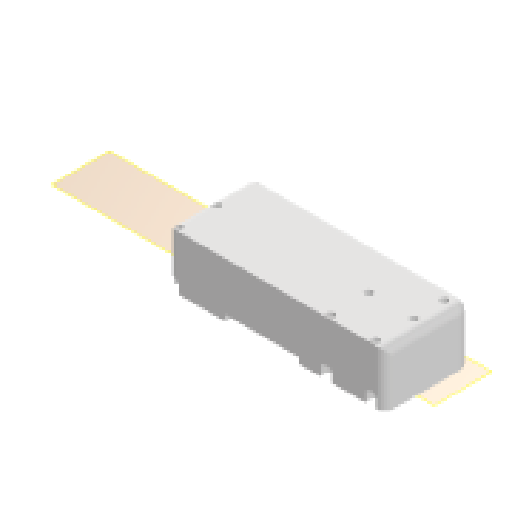
# Autodesk Inventor part: 10_Wellplate_base_Lasercover
Saved by Autodesk Inventor 2024.1 (Build 281209000, 209)
## iProperties
Created: 2024-08-29
Part Number: 10_Wellplate_base_Lasercover
Material: Generisch
Document SubType Name: Modeling
Designer: diederichbenedict
Density: 1 g/cm^3
Appearance: Vorgabe
Author: diederichbenedict
Autodesk Inventor part; units mm, degrees
ref_plane "YZ Plane" through (0, 0, 0) normal (1, 0, 0) x (0, 1, 0)
ref_plane "XZ Plane" through (0, 0, 0) normal (0, 1, 0) x (-1, 0, 0)
ref_plane "XY Plane" through (0, 0, 0) normal (0, 0, 1) x (1, 0, 0)
ref_plane "Arbeitsebene1" through (0, 0, 0) normal (0, 0, 1) x (1, 0, 0)
sketch "Skizze1" plane through (0, 0, 0) normal (0, 0, 1) x (1, 0, 0)
  line L0 (37.9, 26.5) -> (37.9, 13.35) projected
  line L1 (37.9, 13.35) -> (53.9, 13.35) projected
  line L2 (53.9, 13.35) -> (53.9, 13.85) projected
  line L3 (53.9, 13.85) -> (63.9, 13.85) projected
  line L4 (63.9, 13.85) -> (63.9, 27.75) projected
  arc A0 (63.9, 27.75) -> (58.9, 32.75) centre (58.9, 27.75) ccw projected
  line L5 (58.9, 32.75) -> (-58.9, 32.75) projected
  arc A1 (-58.9, 32.75) -> (-63.9, 27.75) centre (-58.9, 27.75) ccw projected
  line L6 (-63.9, 27.75) -> (-63.9, 19.25) projected
  line L7 (-63.9, 19.25) -> (-58.9, 19.25) projected
  line L8 (-58.9, 19.25) -> (-58.9, 19.75) projected
  line L9 (-58.9, 19.75) -> (-38.9, 19.75) projected
  line L10 (-38.9, 19.75) -> (-38.9, 13.85) projected
  line L11 (-38.9, 13.85) -> (-28.9, 13.85) projected
  line L12 (-28.9, 13.85) -> (-28.9, 13.35) projected
  line L13 (-28.9, 13.35) -> (-8.6, 13.35) projected
  line L14 (-8.6, 13.35) -> (-8.6, 26.5) projected
  line L15 (-8.6, 26.5) -> (37.9, 26.5) projected
  circle A2 centre (58.6204, 27.75) radius 1.4 projected
  circle A3 centre (-59.1796, 27.75) radius 1.4 projected
  circle A4 centre (-13.6, 16.25) radius 1.4 projected
  circle A5 centre (-33.6, 16.25) radius 1.4 projected
  circle A6 centre (58.9, 16.25) radius 1.4 projected
  circle A7 centre (42.4, 16.25) radius 1.4 projected
  line L16 (-8.6, -11.9682) -> (-10.6, -13.9682) projected
  line L17 (-8.6, -11.9682) -> (-8.6, 5.15) projected
  line L18 (-8.6, 5.15) -> (-28.9, 5.15) projected
  line L19 (-28.9, 5.15) -> (-28.9, 4.65) projected
  line L20 (-28.9, 4.65) -> (-38.9, 4.65) projected
  line L21 (-38.9, 4.65) -> (-38.9, -1.25) projected
  line L22 (-38.9, -1.25) -> (-58.9, -1.25) projected
  line L23 (-58.9, -1.25) -> (-58.9, -0.75) projected
  line L24 (-58.9, -0.75) -> (-63.9, -0.75) projected
  line L25 (-63.9, -0.75) -> (-63.9, -16.5797) projected
  arc A8 (-49.9, -11.2196) -> (-63.9, -16.5797) centre (-50.2702, -31.2162) ccw projected
  line L26 (-49.9, -11.2196) -> (-49.9, -13.9682) projected
  line L27 (-49.9, -13.9682) -> (-10.6, -13.9682) projected
  circle A9 centre (-13.3796, -11.2637) radius 1.4 projected
  circle A10 centre (-33.6, 2.25) radius 1.4 projected
  circle A11 centre (-13.6, 2.25) radius 1.4 projected
  circle A12 centre (58.6204, -47.75) radius 1.4 projected
  circle A13 centre (58.9, 2.25) radius 1.4 projected
  circle A14 centre (42.4, 2.25) radius 1.4 projected
  circle A15 centre (42.4, -11.2637) radius 1.4 projected
  circle A16 centre (42.4, -31.25) radius 1.4 projected
  line L28 (63.9, 4.65) -> (53.9, 4.65) projected
  line L29 (53.9, 4.65) -> (53.9, 5.15) projected
  line L30 (53.9, 5.15) -> (37.9, 5.15) projected
  line L31 (37.9, 5.15) -> (37.9, -41.35) projected
  line L32 (37.9, -41.35) -> (-33.0276, -41.35) projected
  arc A17 (-59.1255, -49.149) -> (-33.0276, -41.35) centre (-50.2702, -31.2162) ccw projected
  arc A18 (-60.3777, -48.4742) -> (-59.1255, -49.149) centre (-59.1796, -47.75) ccw projected
  arc A19 (-63.9, -45.8527) -> (-60.3777, -48.4742) centre (-50.2702, -31.2162) ccw projected
  line L33 (-63.9, -45.8527) -> (-63.9, -47.75) projected
  arc A20 (-63.9, -47.75) -> (-58.9, -52.75) centre (-58.9, -47.75) ccw projected
  line L34 (-58.9, -52.75) -> (58.9, -52.75) projected
  arc A21 (58.9, -52.75) -> (63.9, -47.75) centre (58.9, -47.75) ccw projected
  line L35 (63.9, -47.75) -> (63.9, 4.65) projected
  line L36 (-16.1, 32.75) -> (63.9, 32.75)
  line L37 (63.9, 32.75) -> (63.9, 0.75)
  line L38 (63.9, 0.75) -> (-16.1, 0.75)
  line L39 (-16.1, 0.75) -> (-16.1, 32.75)
  point P0 (0, 0)
  dimension "d0" = 80
  dimension "d1" = 0
  dimension "d2" = 32
  constraints: 8 end point, 2 parallel, 1 horizontal, 1 perpendicular, 1 point on line
  measures "d0" distance between parallel lines of L4 L39
  measures "d1" distance between parallel lines of L5 L36
  measures "d2" distance between parallel lines of L38 L36
extrude "Extrusion1" add sketch "Skizze1" along normal blind 20 contours L15 L14 L13 L39 L5 A0 L4 L3 L2 L1 L0 | L0 L1 L2 L3 L37 L28 L29 L30 L31 L38 L17 L18 L39 L13 L14 L15 | L18 L17 L38 L39 | L35 L38 L31 L30 L29 L28
fillet "Rundung1" radius 3 9 edges at (62.4355, 31.2855, 20) (63.9, 20.8, 20) (63.9, 9.25, 20) (63.9, 2.7, 20) (21.4, 32.75, 20) (-16.1, 16.75, 20) (-16.1, 0.75, 10) (-16.1, 32.75, 10) (63.9, 0.75, 10)
sketch "Skizze2" plane through (0, 0, 0) normal (0, 0, -1) x (-1, 0, 0)
  arc A0 (13.1, 0.75) -> (16.1, 3.75) centre (13.1, 3.75) ccw projected
  line L0 (16.1, 29.75) -> (16.1, 3.75) projected
  arc A1 (16.1, 29.75) -> (13.1, 32.75) centre (13.1, 29.75) ccw projected
  line L1 (-58.9, 32.75) -> (13.1, 32.75) projected
  arc A2 (-58.9, 32.75) -> (-63.9, 27.75) centre (-58.9, 27.75) ccw projected
  line L2 (-63.9, 3.75) -> (-63.9, 27.75) projected
  arc A3 (-63.9, 3.75) -> (-60.9, 0.75) centre (-60.9, 3.75) ccw projected
  line L3 (13.1, 0.75) -> (-60.9, 0.75) projected
  circle A4 centre (13.6, 2.25) radius 1.4 projected
  circle A5 centre (-42.4, 2.25) radius 1.4 projected
  circle A6 centre (-58.9, 2.25) radius 1.4 projected
  circle A7 centre (-42.4, 16.25) radius 1.4 projected
  circle A8 centre (-58.9, 16.25) radius 1.4 projected
  circle A9 centre (13.6, 16.25) radius 1.4 projected
  circle A10 centre (-58.6204, 27.75) radius 1.4 projected
  point P0 (0, 0)
hole "Bohrung1" at (58.6204, 27.75, 0) at (42.4, 16.25, 0) at (58.9, 2.25, 0) at (58.9, 16.25, 0) at (42.4, 2.25, 0) at (-13.6, 2.25, 0) at (-13.6, 16.25, 0) direction (0, 0, 1) diameter 4.9 depth 4 tip angle 118
sketch "Skizze3" plane through (0, 0, 0) normal (0, 0, -1) x (-1, 0, 0)
  arc A0 (15.9692, 2.8739) -> (11.6629, 0.75) centre (13.6, 2.25) ccw projected
  arc A1 (15.9692, 2.8739) -> (16.1, 3.75) centre (13.1, 3.75) ccw projected
  line L0 (16.1, 29.75) -> (16.1, 3.75) projected
  arc A2 (16.1, 29.75) -> (13.1, 32.75) centre (13.1, 29.75) ccw projected
  line L1 (-58.9, 32.75) -> (13.1, 32.75) projected
  arc A3 (-58.9, 32.75) -> (-63.9, 27.75) centre (-58.9, 27.75) ccw projected
  line L2 (-63.9, 3.75) -> (-63.9, 27.75) projected
  arc A4 (-63.9, 3.75) -> (-60.9, 0.75) centre (-60.9, 3.75) ccw projected
  line L3 (-60.8371, 0.75) -> (-60.9, 0.75) projected
  arc A5 (-56.9629, 0.75) -> (-60.8371, 0.75) centre (-58.9, 2.25) ccw projected
  line L4 (-44.3371, 0.75) -> (-56.9629, 0.75) projected
  arc A6 (-40.4629, 0.75) -> (-44.3371, 0.75) centre (-42.4, 2.25) ccw projected
  line L5 (11.6629, 0.75) -> (-40.4629, 0.75) projected
  circle A7 centre (-58.6204, 27.75) radius 2.45 projected
  circle A8 centre (-42.4, 16.25) radius 2.45 projected
  circle A9 centre (-58.9, 16.25) radius 2.45 projected
  circle A10 centre (13.6, 16.25) radius 2.45 projected
  arc A11 (-58.9, 31.2519) -> (-62.4019, 27.75) centre (-58.9, 27.75) ccw
  line L6 (-58.9, 31.2519) -> (13.1, 31.2519)
  arc A12 (14.6019, 29.75) -> (13.1, 31.2519) centre (13.1, 29.75) ccw
  line L7 (14.6019, 29.75) -> (14.6019, 6.0689)
  arc A13 (14.6019, 6.0689) -> (9.6519, 2.2481) centre (13.6, 2.25) ccw
  line L8 (9.6519, 2.2481) -> (-38.4519, 2.2481)
  arc A14 (-38.4519, 2.2481) -> (-46.3481, 2.2481) centre (-42.4, 2.25) ccw
  line L9 (-46.3481, 2.2481) -> (-54.9519, 2.2481)
  arc A15 (-54.9519, 2.2481) -> (-62.3327, 4.2005) centre (-58.9, 2.25) ccw
  arc A16 (-62.4019, 3.75) -> (-62.3327, 4.2005) centre (-60.9, 3.75) ccw
  line L10 (-62.4019, 3.75) -> (-62.4019, 27.75)
  circle A17 centre (-58.9, 16.25) radius 3.4626
  circle A18 centre (-58.6204, 27.75) radius 3.6913
  circle A19 centre (-42.4, 16.25) radius 3.7166
  circle A20 centre (13.6, 16.25) radius 4.3613
  point P0 (0, 0)
  point P1 (-57.4529, 31.2519)
  point P2 (-61.1978, 30.3926)
  point P3 (-61.3491, 2.3169)
  point P4 (-59.6499, 4.5824)
  point P5 (-61.7336, 4.9993)
  point P6 (14.6019, 12.0053)
  point P7 (14.6019, 20.4947)
  constraints: 12 point on circle, 10 centre point, 10 end point, 10 other
extrude "Extrusion2" cut sketch "Skizze3" against normal blind 18 contours L7 A13 L8 A14 L9 A15 A16 A5 L10 A11 A18 L6 A12 A20
sketch "Skizze4" plane through (-13.1, 0.75, 20) normal (0, -1, 0) x (1, 0, 0)
  circle A0 centre (31.7066, -26.8441) radius 6 projected
  line L0 (45.2066, -35.8441) -> (18.2066, -35.8441)
  line L1 (18.2066, -35.8441) -> (18.2066, -17.8441)
  line L2 (18.2066, -17.8441) -> (45.2066, -17.8441)
  line L3 (45.2066, -17.8441) -> (45.2066, -35.8441)
  line L4 (45.2066, -35.8441) -> (18.2066, -17.8441) construction
  line L5 (18.2066, -35.8441) -> (45.2066, -17.8441) construction
  point P0 (13.1, -20)
  dimension "d15" = 27
  dimension "d16" = 18
  constraints: 12 end point, 2 midpoint, 2 parallel, 1 horizontal, 1 perpendicular
  measures "d15" distance of L1.end L2.end
  measures "d16" distance of L0.end L1.end
extrude "Extrusion3" cut sketch "Skizze4" against normal blind 18 contours A0 | L0 L1 L2 L3
